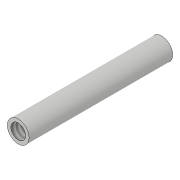
# Autodesk Inventor part: .825in Rod
Saved by Autodesk Inventor 2018.3 (Build 223284000, 284)
## iProperties
Created: 2019-04-08
Part Number: .825in Rod
Material: Generic
Document SubType Name: Modeling
Designer: aye06091
Mass: 0.0891917 g
Surface Area: 3.59661 cm^2
Volume: 0.0891917 cm^3
Density: 1 g/cm^3
Appearance: Default
Author: aye06091
Autodesk Inventor part; units mm, degrees
ref_plane "YZ Plane" through (0, 0, 0) normal (1, 0, 0) x (0, 1, 0)
ref_plane "XZ Plane" through (0, 0, 0) normal (0, 1, 0) x (-1, 0, 0)
ref_plane "XY Plane" through (0, 0, 0) normal (0, 0, 1) x (1, 0, 0)
sketch "Sketch1" plane through (0, 0, 0) normal (0, 0, 1) x (1, 0, 0)
  circle A0 centre (0, 0) radius 1.5875
  dimension "d0" = 3.175
  constraints: 1 centre point
  measures "d0" diameter of A0
extrude "Extrusion1" add sketch "Sketch1" against normal blind 20.955
hole "Hole1" at (0, 0, 0) direction (0, 0, -1) diameter 2.159 end through all
body "Solid1"
